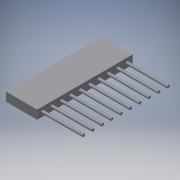
# Autodesk Inventor part: 00_electricpin_2.54_10x
Saved by Autodesk Inventor 2019.4 (Build 234330000, 330)
## iProperties
Created: 2021-10-01
Part Number: 00_electricpin_2.54_10x
Material: Generic
Document SubType Name: Modeling
Designer: diederichbenedict
Density: 1 g/cm^3
Appearance: Default
Author: diederichbenedict
Autodesk Inventor part; units mm, degrees
ref_plane "YZ Plane" through (0, 0, 0) normal (1, 0, 0) x (0, 1, 0)
ref_plane "XZ Plane" through (0, 0, 0) normal (0, 1, 0) x (-1, 0, 0)
ref_plane "XY Plane" through (0, 0, 0) normal (0, 0, 1) x (1, 0, 0)
sketch "Sketch1" plane through (0, 0, 0) normal (1, 0, 0) x (0, 1, 0)
  line L0 (-1.185, -12.92) -> (1.185, -12.92)
  line L1 (1.185, -12.92) -> (1.185, 12.92)
  line L2 (1.185, 12.92) -> (-1.185, 12.92)
  line L3 (-1.185, 12.92) -> (-1.185, -12.92)
  line L4 (-1.185, -12.92) -> (1.185, 12.92) construction
  line L5 (1.185, -12.92) -> (-1.185, 12.92) construction
  point P0 (0, 0)
  dimension "d0" = 2.37
  dimension "d1" = 25.84
  constraints: 12 end point, 2 midpoint, 2 parallel, 1 horizontal, 1 perpendicular
  measures "d0" distance of L2.end L1.end
  measures "d1" distance of L1.end L0.end
extrude "Extrusion1" add sketch "Sketch1" along normal blind 8.43
sketch "Sketch2" plane through (8.43, 0, 0) normal (1, 0, 0) x (0, 0, -1)
  line L0 (12.92, -1.185) -> (12.92, 1.185) projected
  line L1 (12.92, 1.185) -> (-12.92, 1.185) projected
  line L2 (-12.92, 1.185) -> (-12.92, -1.185) projected
  line L3 (-12.92, -1.185) -> (12.92, -1.185) projected
  circle A0 centre (-11.47, 0) radius 0.375
  point P0 (0, 0)
  dimension "d4" = 0.75
  dimension "d5" = 1.45
  constraints: 1 centre point
  measures "d4" diameter of A0
  measures "d5" distance from line of A0.centre L2
extrude "Extrusion2" add sketch "Sketch2" along normal blind 11.15 contours A0
sketch "Sketch3" plane through (0, 0, 0) normal (-1, 0, 0) x (0, 0, 1)
  circle A0 centre (11.47, 0) radius 0.375 projected
  point P0 (0, 0)
extrude "Extrusion3" cut sketch "Sketch3" against normal blind 7
pattern_linear "Rectangular Pattern1" count 10 spacing 2.54 along (0, 0, -1) of "Extrusion2", "Extrusion3"
body "Solid1"
